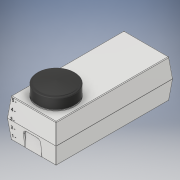
# Autodesk Inventor part: SP0005-FT
Saved by Autodesk Inventor 2019 (Build 230136000, 136)
## iProperties
Created: 2020-09-26
Part Number: SP0005-FT
Material: Polyethylene, High Density
Description: TANK; RECTANGULAR; 5 GAL; 22.00 IN L; 9.25 IN W; 9.77 IN H
Vendor: PLASTIC-MART
Document SubType Name: Modeling
Designer: J. LENDI
Engineer: J. LENDI
Stock Number: SP005-RT
Mass: 2721.55 g
Surface Area: 5473.78 cm^2
Volume: 23866.5 cm^3
Density: 0.114032 g/cm^3
Appearance: Smooth - White
Engr Approved By: J. LENDI
Catalog Web Link: https://www.plastic-mart.com/product/2465/5-gallon-rectangle-flat-bottom-tank-sp0005-rt
Author: J. LENDI
Revision Number: A
Autodesk Inventor part; units mm, degrees
note: some values were not read from the file. Chosen so that the rebuilt part matches the saved one: direction of "Emboss1".
ref_plane "XZ Plane" through (0, 0, 0) normal (0, 1, 0) x (-1, 0, 0)
sketch "Sketch1" plane through (0, 0, 0) normal (0, 0, 1) x (1, 0, 0)
  line L0 (-117.475, -90.424) -> (117.475, -90.424) construction
  line L1 (117.475, -90.424) -> (117.475, 90.424) construction
  line L2 (117.475, 90.424) -> (-117.475, 90.424) construction
  line L3 (-117.475, 90.424) -> (-117.475, -90.424) construction
  line L4 (-117.475, -90.424) -> (117.475, 90.424) construction
  line L5 (117.475, -90.424) -> (-117.475, 90.424) construction
  line L6 (0, 90.424) -> (0, -90.424) construction
  line L7 (-117.475, 0) -> (-107.9711, -90.424)
  line L8 (-117.475, 0) -> (-107.9711, 90.424)
  line L9 (117.475, 0) -> (107.9711, -90.424)
  line L10 (117.475, 0) -> (107.9711, 90.424)
  line L11 (-107.9711, 90.424) -> (107.9711, 90.424)
  line L12 (-107.9711, -90.424) -> (107.9711, -90.424)
  point P0 (0, 0)
  dimension "d4" = 234.95
  dimension "d5" = 180.848
  dimension "d6" = 6
  dimension "d7" = 6
  constraints: 26 end point, 5 midpoint, 3 symmetric about line, 2 horizontal, 2 parallel, 2 point on line, 1 collinear, 1 perpendicular
  measures "d4" distance of L0.start L0.end
  measures "d5" distance of L0.end L1.end
  measures "d6" angle of L3 L8
  measures "d7" angle of L3 L7
extrude "Extrusion1" add sketch "Sketch1" along normal mid plane 558.8
ref_plane "Work Plane1" through (117.475, 0, 0) normal (1, 0, 0) x (0, 1, 0)
sketch "Sketch3" plane through (117.475, 0, 0) normal (1, 0, 0) x (0, 1, 0)
  line L0 (90.424, -279.4) -> (90.424, 279.4) construction
  line L1 (0, 279.4) -> (90.424, 279.4) construction
  line L2 (0, -279.4) -> (0, 279.4) construction
  line L3 (90.424, -279.4) -> (0, -279.4) construction
  line L4 (0, -279.4) -> (0, 279.4) construction
  line L5 (-90.424, 279.4) -> (0, 279.4) construction
  line L6 (-90.424, -279.4) -> (-90.424, 279.4) construction
  line L7 (0, -279.4) -> (-90.424, -279.4) construction
  line L8 (0, 279.4) -> (90.424, 279.4) projected
  line L9 (0, 279.4) -> (90.424, 269.8961)
  line L10 (90.424, -279.4) -> (90.424, 279.4) projected
  line L11 (90.424, 269.8961) -> (90.424, 279.4)
  line L12 (90.424, 279.4) -> (0, 279.4)
  line L13 (0, 279.4) -> (-90.424, 279.4)
  line L14 (0, 279.4) -> (-90.424, 279.4) projected
  line L15 (0, 279.4) -> (-90.424, 269.8961)
  line L16 (-90.424, -279.4) -> (-90.424, 279.4) projected
  line L17 (-90.424, 269.8961) -> (-90.424, 279.4)
  line L18 (90.424, 0) -> (-90.424, 0) construction
  line L19 (0, -279.4) -> (90.424, -279.4) construction
  line L20 (-90.424, -279.4) -> (0, -279.4) construction
  line L21 (0, -279.4) -> (90.424, -279.4)
  line L22 (0, -279.4) -> (90.424, -269.8961)
  line L23 (90.424, -269.8961) -> (90.424, -279.4)
  line L24 (90.424, -279.4) -> (0, -279.4)
  line L25 (0, -279.4) -> (-90.424, -279.4)
  line L26 (0, -279.4) -> (-90.424, -279.4)
  line L27 (0, -279.4) -> (-90.424, -269.8961)
  line L28 (-90.424, -269.8961) -> (-90.424, -279.4)
  point P0 (0, 0)
  dimension "d13" = 6
  dimension "d14" = 6
  constraints: 34 end point, 4 symmetric about line, 2 collinear, 2 midpoint, 2 point on line, 1 perpendicular, 1 vertical
  measures "d13" angle of L1 L9
  measures "d14" angle of L5 L15
extrude "Extrusion2" cut sketch "Sketch3" against normal through all contours L9 L10 L22 L27 L16 L15 keep common part
sketch "Sketch7" plane through (0, 0, 0) normal (1, 0, 0) x (0, 1, 0)
  line L0 (90.424, -269.8961) -> (90.424, 269.8961) projected
  line L1 (90.424, -269.8961) -> (90.424, 269.8961) projected
  line L2 (90.424, 250.8461) -> (157.734, 250.8461) construction
  line L3 (157.734, 250.8461) -> (157.734, 73.0461) construction
  line L4 (157.734, 73.0461) -> (90.424, 73.0461) construction
  line L5 (90.424, 73.0461) -> (90.424, 250.8461) construction
  line L6 (90.424, 250.8461) -> (157.734, 73.0461) construction
  line L7 (157.734, 250.8461) -> (90.424, 73.0461) construction
  line L8 (157.734, 161.9461) -> (90.424, 161.9461) construction
  line L9 (145.034, 250.8461) -> (145.034, 242.5911)
  line L10 (145.034, 250.8461) -> (96.774, 250.8461)
  line L11 (96.774, 250.8461) -> (96.774, 247.6711)
  line L12 (96.774, 247.6711) -> (93.599, 247.6711)
  line L13 (93.599, 247.6711) -> (93.599, 250.8461)
  line L14 (93.599, 250.8461) -> (90.424, 250.8461)
  line L15 (90.424, 250.8461) -> (90.424, 161.9461)
  line L16 (145.034, 73.0461) -> (145.034, 79.3961) construction
  line L17 (145.034, 242.5911) -> (148.209, 242.5911)
  line L18 (145.034, 79.3961) -> (148.209, 79.3961) construction
  arc A0 (157.734, 161.9461) -> (148.209, 242.5911) centre (-514.4228, 123.4425) ccw
  line L19 (157.734, 161.9461) -> (90.424, 161.9461)
  point P0 (0, 0)
  point P1 (124.079, 161.9461)
  dimension "d36" = 107.95
  dimension "d37" = 177.8
  dimension "d38" = 67.31
  dimension "d39" = 12.7
  dimension "d40" = 8.255
  dimension "d41" = 3.175
  dimension "d42" = 3.175
  dimension "d43" = 3.175
  dimension "d44" = 6.35
  dimension "d45" = 3.175
  dimension "d46" = 3.175
  dimension "d47" = 673.2587
  constraints: 36 end point, 6 point on line, 4 horizontal, 4 midpoint, 4 perpendicular, 2 collinear, 2 parallel, 2 point on circle, 2 vertical, 1 centre point
  measures "d36" vertical distance of L0.end point (124.079, 161.946)
  measures "d37" distance of L2.end L3.end
  measures "d38" distance between parallel lines of L0 L3
  measures "d39" distance between parallel lines of L3 L9
  measures "d40" distance of L9.start L9.end
  measures "d41" distance between parallel lines of L12 L10
  measures "d42" distance of L11.end L12.end
  measures "d43" distance between parallel lines of L15 L13
  measures "d44" distance of L16.start L16.end
  measures "d45" distance of L9.end L17.end
  measures "d46" distance of L16.end L18.end
  measures "d47" radius of A0
revolve "Revolution1" add sketch "Sketch7" angle 360 about axis through (0, 157.734, 161.9461) along (0, -1, 0)
ref_plane "Work Plane4" through (0, 0, 279.4) normal (0, 0, 1) x (1, 0, 0)
sketch "Sketch8" plane through (0, 0, 279.4) normal (0, 0, 1) x (1, 0, 0)
  line L0 (-107.9711, -90.424) -> (107.9711, -90.424) projected
  line L1 (-38.1, -90.424) -> (38.1, -90.424)
  line L2 (38.1, -90.424) -> (38.1, -26.924)
  line L3 (25.4, -14.224) -> (-25.4, -14.224)
  line L4 (-38.1, -26.924) -> (-38.1, -90.424)
  line L5 (0, 207.3656) -> (0, -140.0556) projected
  arc A0 (-25.4, -14.224) -> (-38.1, -26.924) centre (-25.4, -26.924) ccw
  arc A1 (38.1, -26.924) -> (25.4, -14.224) centre (25.4, -26.924) ccw
  point P0 (0, 0)
  dimension "d52" = 76.2
  dimension "d53" = 76.2
  dimension "d54" = 38.1
  dimension "d55" = 12.7
  constraints: 8 end point, 4 point on circle, 4 tangent, 2 centre point, 2 parallel, 1 equal radius, 1 horizontal, 1 perpendicular, 1 point on line
  measures "d52" distance between parallel lines of L2 L4
  measures "d53" distance between parallel lines of L0 L3
  measures "d54" distance between parallel lines of L5 L4
  measures "d55" radius of A0
extrude "Extrusion5" cut sketch "Sketch8" against normal blind 9.4996
fillet "Fillet1" radius 3.175 24 edges at (107.9711, 90.424, 0) (0, 90.424, 269.8961) (112.723, 45.212, 274.648) (112.723, -45.212, 274.648) (107.9711, -90.424, 0) (0, -90.424, 269.8961) (112.723, 45.212, -274.648) (112.723, -45.212, -274.648) (-112.723, 45.212, -274.648) (0, 90.424, -269.8961) (-112.723, -45.212, -274.648) (0, -90.424, -269.8961) (-107.9711, -90.424, 0) (-107.9711, 90.424, 0) (-117.475, 0, 0) (-112.723, 45.212, 274.648) (-112.723, -45.212, 274.648) (117.475, 0, 0) (0, 145.034, 73.0461) (34.3803, -17.9437, 277.514) (38.1, -58.6533, 273.2353) (-34.3803, -17.9437, 277.514) (-38.1, -58.6533, 273.2353) (0, -14.224, 277.905)
sketch "Sketch9" plane through (0, 0, 279.4) normal (0, 0, 1) x (1, 0, 0)
  line L0 (-101.6, 85.344) -> (-63.5, 85.344) construction
  line L1 (-63.5, 85.344) -> (-63.5, -79.756) construction
  line L2 (-63.5, -79.756) -> (-101.6, -79.756) construction
  line L3 (-101.6, -79.756) -> (-101.6, 85.344) construction
  line L4 (105.1123, 90.424) -> (-105.1123, 90.424) projected
  line L5 (0, 207.3656) -> (0, -140.0556) projected
  line L6 (-100.8643, 76.1384) -> (-99.2284, 76.274)
  spline S0 degree 2 poles (-99.2284, 76.274) (-99.0445, 75.0736) (-97.728, 73.8733) (-96.7891, 73.8733) knots 0 0 0 1 2 2 2
  spline S1 degree 2 poles (-96.7891, 73.8733) (-95.6469, 73.8733) (-94.0981, 75.577) (-94.0981, 76.9806) knots 0 0 0 1 2 2 2
  spline S2 degree 2 poles (-94.0981, 76.9806) (-94.0981, 78.3164) (-95.5888, 79.8652) (-96.8085, 79.8652) knots 0 0 0 1 2 2 2
  spline S3 degree 2 poles (-96.8085, 79.8652) (-97.5635, 79.8652) (-98.7735, 79.1779) (-99.122, 78.6262) knots 0 0 0 1 2 2 2
  line L7 (-99.122, 78.6262) -> (-100.5836, 78.8198)
  line L8 (-100.5836, 78.8198) -> (-99.3543, 85.344)
  line L9 (-99.3543, 85.344) -> (-93.043, 85.344)
  line L10 (-93.043, 85.344) -> (-93.043, 83.8533)
  line L11 (-93.043, 83.8533) -> (-98.1056, 83.8533)
  line L12 (-98.1056, 83.8533) -> (-98.7928, 80.446)
  spline S4 degree 2 poles (-98.7928, 80.446) (-97.6506, 81.2397) (-96.3922, 81.2397) knots 0 0 0 1 1 1
  spline S5 degree 2 poles (-96.3922, 81.2397) (-94.7273, 81.2397) (-92.4428, 78.9359) (-92.4428, 77.1258) knots 0 0 0 1 2 2 2
  spline S6 degree 2 poles (-92.4428, 77.1258) (-92.4428, 75.3931) (-93.4495, 74.1347) knots 0 0 0 1 1 1
  spline S7 degree 2 poles (-93.4495, 74.1347) (-94.6692, 72.5956) (-96.7794, 72.5956) knots 0 0 0 1 1 1
  spline S8 degree 2 poles (-96.7794, 72.5956) (-98.5121, 72.5956) (-100.7095, 74.5316) (-100.8643, 76.1384) knots 0 0 0 1 2 2 2
  line L13 (-86.2574, 76.6224) -> (-86.2574, 78.1906)
  line L14 (-86.2574, 78.1906) -> (-81.4562, 78.1906)
  line L15 (-81.4562, 78.1906) -> (-81.4562, 76.6224)
  line L16 (-81.4562, 76.6224) -> (-86.2574, 76.6224)
  line L17 (-95.8695, 36.2466) -> (-95.8695, 39.2861)
  line L18 (-95.8695, 39.2861) -> (-101.3774, 39.2861)
  line L19 (-101.3774, 39.2861) -> (-101.3774, 40.7187)
  line L20 (-101.3774, 40.7187) -> (-95.5888, 48.9466)
  line L21 (-95.5888, 48.9466) -> (-94.3111, 48.9466)
  line L22 (-94.3111, 48.9466) -> (-94.3111, 40.7187)
  line L23 (-94.3111, 40.7187) -> (-92.5977, 40.7187)
  line L24 (-92.5977, 40.7187) -> (-92.5977, 39.2861)
  line L25 (-92.5977, 39.2861) -> (-94.3111, 39.2861)
  line L26 (-94.3111, 39.2861) -> (-94.3111, 36.2466)
  line L27 (-94.3111, 36.2466) -> (-95.8695, 36.2466)
  line L28 (-95.8695, 40.7187) -> (-95.8695, 46.4492)
  line L29 (-95.8695, 46.4492) -> (-99.8479, 40.7187)
  line L30 (-99.8479, 40.7187) -> (-95.8695, 40.7187)
  line L31 (-86.2574, 40.0605) -> (-86.2574, 41.6286)
  line L32 (-86.2574, 41.6286) -> (-81.4562, 41.6286)
  line L33 (-81.4562, 41.6286) -> (-81.4562, 40.0605)
  line L34 (-81.4562, 40.0605) -> (-86.2574, 40.0605)
  line L35 (-100.8546, 3.0533) -> (-99.2962, 3.2566)
  spline S9 degree 2 poles (-99.2962, 3.2566) (-99.0252, 1.9304) (-97.7377, 0.7591) (-96.8085, 0.7591) knots 0 0 0 1 2 2 2
  spline S10 degree 2 poles (-96.8085, 0.7591) (-95.705, 0.7591) (-94.1949, 2.2886) (-94.1949, 3.4114) knots 0 0 0 1 2 2 2
  spline S11 degree 2 poles (-94.1949, 3.4114) (-94.1949, 4.4859) (-95.5985, 5.8798) (-96.6826, 5.8798) knots 0 0 0 1 2 2 2
  spline S12 degree 2 poles (-96.6826, 5.8798) (-97.1182, 5.8798) (-97.7764, 5.7056) knots 0 0 0 1 1 1
  line L36 (-97.7764, 5.7056) -> (-97.6119, 7.0704)
  spline S13 degree 2 poles (-97.6119, 7.0704) (-97.4473, 7.0511) (-97.3602, 7.0511) knots 0 0 0 1 1 1
  spline S14 degree 2 poles (-97.3602, 7.0511) (-96.3632, 7.0511) (-94.766, 8.0965) (-94.766, 9.171) knots 0 0 0 1 2 2 2
  spline S15 degree 2 poles (-94.766, 9.171) (-94.766, 10.0325) (-95.9276, 11.1553) (-96.8472, 11.1553) knots 0 0 0 1 2 2 2
  spline S16 degree 2 poles (-96.8472, 11.1553) (-97.7571, 11.1553) (-98.9671, 10.0131) (-99.1413, 8.8612) knots 0 0 0 1 2 2 2
  line L37 (-99.1413, 8.8612) -> (-100.6998, 9.1419)
  spline S17 degree 2 poles (-100.6998, 9.1419) (-100.4094, 10.7101) (-98.3863, 12.4331) (-96.8762, 12.4331) knots 0 0 0 1 2 2 2
  spline S18 degree 2 poles (-96.8762, 12.4331) (-95.8405, 12.4331) (-94.0884, 11.5425) (-93.1591, 10.0034) (-93.1591, 9.1419) knots 0 0 0 1 2 3 3 3
  spline S19 degree 2 poles (-93.1591, 9.1419) (-93.1591, 8.3191) (-94.04, 6.964) (-94.9112, 6.5671) knots 0 0 0 1 2 2 2
  spline S20 degree 2 poles (-94.9112, 6.5671) (-93.7787, 6.3057) (-92.5396, 4.6698) (-92.5396, 3.4405) knots 0 0 0 1 2 2 2
  spline S21 degree 2 poles (-92.5396, 3.4405) (-92.5396, 1.7852) (-94.9693, -0.5283) (-96.8181, -0.5283) knots 0 0 0 1 2 2 2
  spline S22 degree 2 poles (-96.8181, -0.5283) (-98.4928, -0.5283) (-100.6998, 1.4658) (-100.8546, 3.0533) knots 0 0 0 1 2 2 2
  line L38 (-86.2574, 3.4986) -> (-86.2574, 5.0667)
  line L39 (-86.2574, 5.0667) -> (-81.4562, 5.0667)
  line L40 (-81.4562, 5.0667) -> (-81.4562, 3.4986)
  line L41 (-81.4562, 3.4986) -> (-86.2574, 3.4986)
  line L42 (-92.6752, -35.3769) -> (-92.6752, -36.8773)
  line L43 (-92.6752, -36.8773) -> (-101.0676, -36.8773)
  spline S23 degree 2 poles (-101.0676, -36.8773) (-101.087, -36.3158) (-100.8837, -35.7931) knots 0 0 0 1 1 1
  spline S24 degree 2 poles (-100.8837, -35.7931) (-100.5643, -34.9316) (-99.151, -33.2763) (-97.8152, -32.1825) knots 0 0 0 1 2 2 2
  spline S25 degree 2 poles (-97.8152, -32.1825) (-95.7534, -30.4789) (-94.3014, -28.5042) (-94.3014, -27.6136) knots 0 0 0 1 2 2 2
  spline S26 degree 2 poles (-94.3014, -27.6136) (-94.3014, -26.6843) (-95.6275, -25.4163) (-96.6923, -25.4163) knots 0 0 0 1 2 2 2
  spline S27 degree 2 poles (-96.6923, -25.4163) (-97.8152, -25.4163) (-99.1607, -26.7715) (-99.1704, -27.9621) knots 0 0 0 1 2 2 2
  line L44 (-99.1704, -27.9621) -> (-100.7772, -27.7975)
  spline S28 degree 2 poles (-100.7772, -27.7975) (-100.6127, -26.0068) (-98.4637, -24.1289) (-96.6536, -24.1289) knots 0 0 0 1 2 2 2
  spline S29 degree 2 poles (-96.6536, -24.1289) (-94.8241, -24.1289) (-92.6945, -26.1519) (-92.6945, -27.6523) knots 0 0 0 1 2 2 2
  spline S30 degree 2 poles (-92.6945, -27.6523) (-92.6945, -28.417) (-93.314, -29.8884) (-94.766, -31.5146) (-96.4406, -32.9375) knots 0 0 0 1 2 3 3 3
  spline S31 degree 2 poles (-96.4406, -32.9375) (-97.8442, -34.1088) (-98.638, -34.951) (-98.8993, -35.3769) knots 0 0 0 1 2 2 2
  line L45 (-98.8993, -35.3769) -> (-92.6752, -35.3769)
  line L46 (-86.2574, -33.0634) -> (-86.2574, -31.4952)
  line L47 (-86.2574, -31.4952) -> (-81.4562, -31.4952)
  line L48 (-81.4562, -31.4952) -> (-81.4562, -33.0634)
  line L49 (-81.4562, -33.0634) -> (-86.2574, -33.0634)
  line L50 (-94.9983, -73.4392) -> (-96.5568, -73.4392)
  line L51 (-96.5568, -73.4392) -> (-96.5568, -63.5076)
  spline S32 degree 2 poles (-96.5568, -63.5076) (-97.1182, -64.04) (-98.9477, -65.1145) (-99.6737, -65.3855) knots 0 0 0 1 2 2 2
  line L52 (-99.6737, -65.3855) -> (-99.6737, -63.8755)
  spline S33 degree 2 poles (-99.6737, -63.8755) (-98.3669, -63.2656) (-96.4116, -61.5136) (-96.005, -60.6908) knots 0 0 0 1 2 2 2
  line L53 (-96.005, -60.6908) -> (-94.9983, -60.6908)
  line L54 (-94.9983, -60.6908) -> (-94.9983, -73.4392)
  line L55 (-86.2574, -69.6253) -> (-86.2574, -68.0572)
  line L56 (-86.2574, -68.0572) -> (-81.4562, -68.0572)
  line L57 (-81.4562, -68.0572) -> (-81.4562, -69.6253)
  line L58 (-81.4562, -69.6253) -> (-86.2574, -69.6253)
  point P0 (0, 0)
  dimension "d58" = 5.08
  dimension "d59" = 101.6
  dimension "d60" = 165.1
  dimension "d61" = 38.1
  constraints: 2 other
  measures "d58" distance between parallel lines of L4 L0
  measures "d59" distance between parallel lines of L5 L3
  measures "d60" distance between parallel lines of L2 L0
  measures "d61" distance of L1.end L2.end
emboss "Emboss1" sketch "Sketch9" operation cut depth 2.54 direction (0, 0, -1)
equation "\"d7\" = d6"
equation "\"d14\" = d13"
equation "\"d54\" = 0.5 * d52"
body "Solid1"
